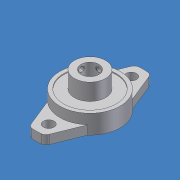
# Autodesk Inventor part: HBR8x
Saved by Autodesk Inventor 2015 (Build 190159000, 159)
## iProperties
Category: PARTsolutions
Created: 2015-02-25
Part Number: HBR8x
Catalog Web Link: www.cadenas.de
Description: HBT, HBR, HBRS, HBRSX x - Ball Bearing Units - Rhomb Flanged Type
Document SubType Name: Modeling
Designer: PARTsolutions
Material: Generic
Density: 1 g/cm^3
Appearance: RGB(192,192,192)
NB: HBR8x
NN: HBT, HBR, HBRS, HBRSX x
NT: Ball Bearing Units - Rhomb Flanged Type
NBSYN: $PN.x
LINA: HBR8x
PN: HBR8
TYPE: HBR
TS: R
MATALG: '','Steel'
MATH: Zinc Alloy Die Cast
MATB: 52100 Bearing Steel
MATRS: Nitrile Rubber (NBR)
MATSS: 4137 Alloy Steel
MATER: 1020 Steel
STER: Black Oxide
PRECISION: JIS B 1558/JIS B 1559
OT: -10 ~+ 80
D: 8
L: 48
L1: 37
TT: 4.0
A2: 4.5
A1: 8.5
DD: 4.8
W: 27
A: 16.0
A11: 16.0
A22: 16.0
B: 15.0
B1: 15.0
B2: 15.0
S: 3.5
CR1: 3300
CR2: -
COR1: 1260
COR2: -
W1: -
W2: 30
W3: -
MASS: 30
CR: 3300
COR: 1260
D1: 14.000
M1: -
M2: M3 x 0.5
TT1: 0
TT2: 0.59
ALC1: 0
ALC2: 0.39
MMAX1: 0.000
MMAX2: 3.000
M: M3 x 0.5
T: 0.59
ALC: 0.39
MMAX: 3.000
TSALG: 'R', 'Eccentric Ring'
X: 2.000
DS: 3.000
LS: 3.000
DS1: 0.000
LS1: 0.000
DS2: 3.000
LS2: 3.000
KT: DUMMY
SUPPLIER: CATALOGS*MISUMI
ARTICLENO: HBR8x
BOMINFO: HBR8x
CREATOR: CADENAS GmbH
PSOL_IDENT_0: {\\10.0.0.236\data_v8\23d-libs\misumi\metric\12_bearing_holders\hbt.prj},175 {VTYP=3D},{NB=HBR8x},{L
PSOL_IDENT_1: INA=HBR8x},{NN=HBT, HBR, HBRS, HBRSX x},{DATE=21.11.2014 02:48:57},{GEOMDATE=07.10.2008 10:42:00},{V
PSOL_IDENT_2: ERSION=},{LINEID=80},{LINESUBID=-1},{WBVAR=TS,MAT}  {NB=HBR8x},{LINA=HBR8x},{KT=DUMMY},{PN=HBR8},{TY
PSOL_IDENT_3: PE=HBR},{TS=R},{MAT=},{MATALG=    '','Steel'     },{MATH=Zinc Alloy Die Cast},{MATB=52100 Bearing St
PSOL_IDENT_4: eel},{MATRS=Nitrile Rubber (NBR)},{MATSS=4137 Alloy Steel},{MATER=1020 Steel},{STER=Black Oxide},{PR
PSOL_IDENT_5: ECISION=JIS B 1558/JIS B 1559},{OT=-10 ~+ 80},{D=8},{L=48},{L1=37},{TT=4.0},{A2=4.5},{A1=8.5},{DD=4.
PSOL_IDENT_6: 8},{W=27},{A=16.0},{A11=16.0},{A22=16.0},{B=15.0},{B1=15.0},{B2=15.0},{S=3.5},{CR1=3300},{CR2=-},{CO
PSOL_IDENT_7: R1=1260},{COR2=-},{W1=-},{W2=30},{W3=-},{MASS=30},{CR=3300},{COR=1260},{D1=14.000},{M1=-},{M2=M3 x 0
PSOL_IDENT_8: .5},{TT1=0},{TT2=0.59},{ALC1=0},{ALC2=0.39},{MMAX1=0.000},{MMAX2=3.000},{M=M3 x 0.5},{T=0.59},{ALC=0
PSOL_IDENT_9: .39},{MMAX=3},{TSALG='R', 'Eccentric Ring'},{X=2},{DS=3},{LS=3},{DS1=0.000},{LS1=0.000},{DS2=3.000},
PSOL_IDENT_10: {LS2=3.000}
Title: HBR8x
Author: Cadenas PARTsolutions
Comments: Ball Bearing Units - Rhomb Flanged Type
Autodesk Inventor part; units mm, degrees
sketch "Sketch_1" plane through (0, 0, 0) normal (1, 0, 0) x (0, 1, 0)
  line L0 (0, -8) -> (0, 8)
  line L1 (7, 8) -> (4, 8)
  line L2 (4, 8) -> (4, -7)
  line L3 (4, -7) -> (5.6375, -7)
  arc A0 (5.7375, -7) -> (5.6375, -7) centre (5.6875, -7) ccw
  line L4 (5.7375, -7) -> (11.8125, -7)
  line L5 (11.8125, -7) -> (11.8125, -8)
  line L6 (11.8125, -8) -> (24, -8)
  line L7 (24, -8) -> (24, -4)
  line L8 (24, -4) -> (13.5, -4)
  line L9 (13.5, -4) -> (13.5, 0.5)
  line L10 (13.5, 0.5) -> (11.8125, 0.5)
  line L11 (11.8125, 0.5) -> (11.8125, 0)
  line L12 (11.8125, 0) -> (5.6875, 0)
  line L13 (5.6875, 0) -> (5.6875, 0.5)
  line L14 (5.6875, 0.5) -> (7, 0.5)
  line L15 (7, 0.5) -> (7, 8)
  constraints: 32 end point, 2 point on circle, 1 centre point
revolve "Revolution1" add sketch "Sketch_1" angle 360 about axis through (0, 0, -8) along (0, 0, -1)
sketch "Sketch_2" plane through (0, 0, 0) normal (0, 0, 1) x (1, 0, 0)
  line L0 (-54, -96) -> (54, -96)
  line L1 (54, -96) -> (54, 96)
  line L2 (54, 96) -> (-54, 96)
  line L3 (-54, 96) -> (-54, -96)
  arc A0 (-9, 10.0623) -> (-9, -10.0623) centre (0, 0) ccw
  line L4 (-9, -10.0623) -> (-4.0569, -22.3105)
  arc A1 (-4.0569, -22.3105) -> (-1.5531, -24) centre (-1.5531, -21.3) ccw
  line L5 (-1.5531, -24) -> (1.5531, -24)
  arc A2 (1.5531, -24) -> (4.0569, -22.3105) centre (1.5531, -21.3) ccw
  line L6 (4.0569, -22.3105) -> (9, -10.0623)
  arc A3 (9, -10.0623) -> (9, 10.0623) centre (0, 0) ccw
  line L7 (9, 10.0623) -> (4.0569, 22.3105)
  arc A4 (4.0569, 22.3105) -> (1.5531, 24) centre (1.5531, 21.3) ccw
  line L8 (1.5531, 24) -> (-1.5531, 24)
  arc A5 (-1.5531, 24) -> (-4.0569, 22.3105) centre (-1.5531, 21.3) ccw
  line L9 (-4.0569, 22.3105) -> (-9, 10.0623)
  constraints: 20 end point, 12 point on circle, 6 centre point
extrude "Extrusion1" cut sketch "Sketch_2" along normal mid plane 32
sketch "Sketch_3" plane through (0, 0, 0) normal (1, 0, 0) x (0, 1, 0)
  line L0 (18.5, -8) -> (18.5, 8)
  line L1 (18.5, 8) -> (22.34, 8)
  line L2 (22.34, 8) -> (22.34, -4)
  line L3 (22.34, -4) -> (20.9, -4)
  line L4 (20.9, -4) -> (20.9, -8)
  line L5 (20.9, -8) -> (18.5, -8)
  line L6 (18.5, -8) -> (18.5, 8)
  constraints: 14 end point
revolve "Revolution2" cut sketch "Sketch_3" angle 360 about axis through (0, 18.5, -8) along (0, 0, -1)
sketch "Sketch_4" plane through (0, 0, 0) normal (1, 0, 0) x (0, 1, 0)
  line L0 (-18.5, -8) -> (-18.5, 8)
  line L1 (-18.5, 8) -> (-14.66, 8)
  line L2 (-14.66, 8) -> (-14.66, -4)
  line L3 (-14.66, -4) -> (-16.1, -4)
  line L4 (-16.1, -4) -> (-16.1, -8)
  line L5 (-16.1, -8) -> (-18.5, -8)
  line L6 (-18.5, -8) -> (-18.5, 8)
  constraints: 14 end point
revolve "Revolution3" cut sketch "Sketch_4" angle 360 about axis through (0, -18.5, -8) along (0, 0, -1)
sketch "Sketch_5" plane through (0, 0, 0) normal (1, 0, 0) x (0, 1, 0)
  line L0 (3.65, 6) -> (7, 6)
  line L1 (7, 6) -> (7, 4.5)
  line L2 (7, 4.5) -> (6.7295, 4.7705)
  line L3 (6.7295, 4.7705) -> (3.9205, 4.7705)
  line L4 (3.9205, 4.7705) -> (3.65, 4.5)
  line L5 (3.65, 4.5) -> (3.65, 6)
  line L6 (3.65, 6) -> (7, 6)
  constraints: 14 end point
revolve "Revolution4" cut sketch "Sketch_5" angle 360 about axis through (0, 3.65, 6) along (0, -1, 0)
thread "Thread1" size "M3x0.5" class "6H" standard "ISO Metric profile" full length
sketch "Sketch_6" plane through (0, 0, 0) normal (0, 1, 0) x (-1, 0, 0)
  line L0 (7, 6) -> (3.65, 6)
  line L1 (3.65, 6) -> (3.65, 7.5)
  line L2 (3.65, 7.5) -> (3.9205, 7.2295)
  line L3 (3.9205, 7.2295) -> (6.7295, 7.2295)
  line L4 (6.7295, 7.2295) -> (7, 7.5)
  line L5 (7, 7.5) -> (7, 6)
  line L6 (7, 6) -> (3.65, 6)
  constraints: 14 end point
revolve "Revolution5" cut sketch "Sketch_6" angle 360 about axis through (-7, 0, 6) along (-1, 0, 0)
thread "Thread2" size "M3x0.5" class "6H" standard "ISO Metric profile" full length
ref_plane "to_screw_XY" through (0, 4, 6) normal (0, 1, 0) x (1, 0, 0)
ref_plane "to_screw_YZ" through (0, 4, 6) normal (1, 0, 0) x (0, 0, -1)
ref_plane "to_screw_ZX" through (0, 4, 6) normal (0, 0, -1) x (0, 1, 0)
ref_plane "to_screw_2_XY" through (-4, 0, 6) normal (-1, 0, 0) x (0, 0, -1)
ref_plane "to_screw_2_YZ" through (-4, 0, 6) normal (0, 0, -1) x (0, -1, 0)
ref_plane "to_screw_2_ZX" through (-4, 0, 6) normal (0, -1, 0) x (-1, 0, 0)
body "Solid1"
